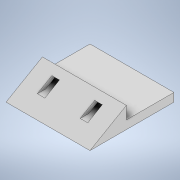
# Autodesk Inventor part: Helenowiak_korpus
Saved by Autodesk Inventor 2021 (Build 250183000, 183)
## iProperties
Created: 2021-03-29
Part Number: Helenowiak_korpus
Material: Ogólny
Document SubType Name: Modeling
Designer: jakub
Density: 1 g/cm^3
Appearance: Domyślna
Author: jakub
Autodesk Inventor part; units mm, degrees
ref_plane "YZ Plane" through (0, 0, 0) normal (1, 0, 0) x (0, 1, 0)
ref_plane "XZ Plane" through (0, 0, 0) normal (0, 1, 0) x (-1, 0, 0)
ref_plane "XY Plane" through (0, 0, 0) normal (0, 0, 1) x (1, 0, 0)
sketch "Szkic1" plane through (0, 0, 0) normal (0, 1, 0) x (-1, 0, 0)
  line L0 (0, 0) -> (-100, 0)
  line L1 (-100, 0) -> (-100, -100)
  line L2 (-100, -100) -> (0, -100)
  line L3 (0, -100) -> (0, 0)
  dimension "d0" = 100
  dimension "d1" = 100
  constraints: 8 end point, 2 parallel, 1 horizontal, 1 perpendicular
  measures "d0" distance of L2.end L1.end
  measures "d1" distance of L1.end L0.end
extrude "Wyciągnięcie proste1" add sketch "Szkic1" along normal blind 10
sketch "Szkic3" plane through (0, 0, -100) normal (-1, 0, 0) x (0, 0, 1)
  line L0 (100, 0) -> (0, 0) projected
  line L1 (100, 0) -> (65.359, 20)
  line L2 (100, 0) -> (140, 0) construction
  line L3 (65.359, 20) -> (65.359, 0)
  line L4 (0, 10) -> (100, 10) projected
  line L5 (100, 0) -> (100, 10) projected
  line L6 (82.6795, 10) -> (100, 10)
  line L7 (100, 10) -> (100, 0)
  line L8 (100, 0) -> (82.6795, 10)
  dimension "d4" = 40
  dimension "d5" = 150
  constraints: 12 end point, 2 horizontal, 2 point on line, 1 equal length, 1 midpoint, 1 perpendicular, 1 vertical
  measures "d4" distance of L0.start L1.end
  measures "d5" angle of L2 L1
extrude "Wyciągnięcie proste2" cut sketch "Szkic3" against normal blind 300 contours L1 L4 L5
sketch "Szkic4" plane through (0, 0, -100) normal (-1, 0, 0) x (0, 0, 1)
  line L0 (0, 10) -> (82.6795, 10) projected
  line L1 (82.6795, 10) -> (56.6987, 25)
  line L2 (82.6795, 10) -> (112.6795, 10) construction
  line L3 (56.6987, 25) -> (56.6987, 10)
  line L4 (82.6795, 10) -> (56.6987, 10)
  point P0 (100, 0)
  dimension "d8" = 30
  dimension "d9" = 150
  constraints: 8 end point, 1 equal length, 1 horizontal, 1 perpendicular, 1 point on line, 1 vertical
  measures "d8" distance of L0.end L1.end
  measures "d9" angle of L2 L1
extrude "Wyciągnięcie proste3" add sketch "Szkic4" against normal blind 10
sketch "Szkic10" plane through (100, 0, -100) normal (1, 0, 0) x (0, 0, -1)
  line L0 (-82.6795, 10) -> (0, 10) projected
  line L1 (0, 10) -> (-56.6987, 10) projected
  line L2 (-82.6795, 10) -> (-56.6987, 10)
  line L3 (-100, 0) -> (-56.6987, 25) projected
  line L4 (-56.6987, 10) -> (-56.6987, 25)
  line L5 (-56.6987, 25) -> (-82.6795, 10)
  constraints: 6 end point, 2 collinear, 1 perpendicular
extrude "Wyciągnięcie proste4" add sketch "Szkic10" against normal blind 10
sketch "Szkic16" plane through (0, 0, 0) normal (0, 0.8660254, 0.5) x (1, 0, 0)
  line L0 (10, 20) -> (90, 20) projected
  line L1 (10, 20) -> (10, 50)
  line L2 (90, 50) -> (90, 42.5) projected
  line L3 (10, 50) -> (90, 50)
  line L4 (90, 20) -> (90, 42.5) projected
  line L5 (90, 50) -> (90, 20)
  line L6 (10, 42.5) -> (10, 20) projected
  line L7 (90, 20) -> (10, 20)
  line L8 (0, 50) -> (10, 50) projected
  line L9 (10, 20) -> (10, 50)
  line L10 (100, 50) -> (90, 50) projected
  line L11 (10, 50) -> (90, 50)
  point P0 (0, 0)
  constraints: 12 end point, 4 perpendicular, 1 collinear, 1 vertical
extrude "Wyciągnięcie proste5" add sketch "Szkic16" against normal blind 5
sketch "Szkic20" plane through (100, 0, -100) normal (0, 0, -1) x (-1, 0, 0)
  line L0 (90, 10) -> (10, 10) projected
  line L1 (20, 10) -> (27, 10)
  line L2 (27, 10) -> (27, 20)
  line L3 (27, 20) -> (20, 20)
  line L4 (20, 20) -> (20, 10)
  point P0 (100, 0)
  dimension "d18" = 7
  dimension "d19" = 10
  constraints: 8 end point, 3 perpendicular, 2 point on line
  measures "d18" distance of L1.start L1.end
  measures "d19" distance of L1.end L2.end
extrude "Wyciągnięcie proste6" cut sketch "Szkic20" against normal blind 146.5
sketch "Szkic21" plane through (100, 0, -100) normal (0, 0, -1) x (-1, 0, 0)
  line L0 (90, 10) -> (27, 10) projected
  line L1 (80, 10) -> (73, 10)
  line L2 (73, 10) -> (73, 20)
  line L3 (73, 20) -> (80, 20)
  line L4 (80, 20) -> (80, 10)
  point P0 (100, 0)
  dimension "d22" = 7
  dimension "d23" = 10
  constraints: 8 end point, 2 perpendicular, 2 point on line, 1 vertical
  measures "d22" distance of L1.start L1.end
  measures "d23" distance of L1.end L2.end
extrude "Wyciągnięcie proste7" cut sketch "Szkic21" against normal blind 115.75
sketch "Szkic22" plane through (100, 0, -100) normal (0, 0, -1) x (-1, 0, 0)
  line L0 (73, 10) -> (73, 20) projected
  line L1 (73, 10) -> (71, 10)
  line L2 (71, 10) -> (71, 20)
  line L3 (71, 20) -> (73, 20)
  line L4 (73, 20) -> (73, 10)
  point P0 (100, 0)
  dimension "d26" = 2
  constraints: 8 end point, 2 parallel, 1 horizontal, 1 perpendicular
  measures "d26" distance of L2.end L3.end
extrude "Wyciągnięcie proste8" cut sketch "Szkic22" against normal blind 92.75
sketch "Szkic23" plane through (100, 0, -100) normal (0, 0, -1) x (-1, 0, 0)
  line L0 (27, 20) -> (27, 10) projected
  line L1 (27, 10) -> (29, 10)
  line L2 (29, 10) -> (29, 20)
  line L3 (29, 20) -> (27, 20)
  line L4 (27, 20) -> (27, 10)
  point P0 (100, 0)
  dimension "d29" = 2
  constraints: 8 end point, 2 parallel, 1 horizontal, 1 perpendicular
  measures "d29" distance of L3.end L2.end
extrude "Wyciągnięcie proste9" cut sketch "Szkic23" against normal blind 244.5
